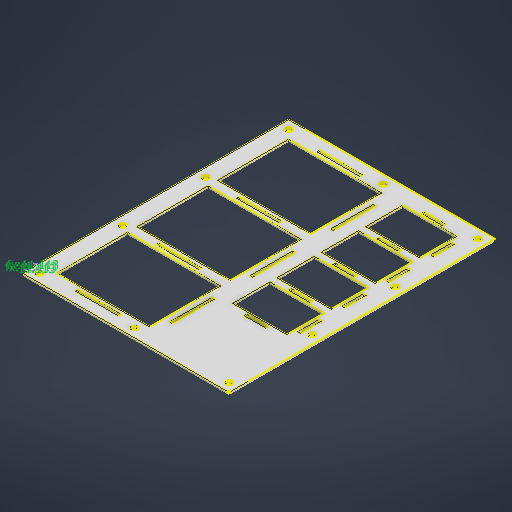
# Autodesk Inventor part: SignFace
Saved by Autodesk Inventor 2026 (Build 300175000, 175)
## iProperties
Created: 2025-05-16
Part Number: SignFace
Material: Generic
Document SubType Name: Modeling
Designer: Riley
Density: 1 g/cm^3
Appearance: Default
Author: Riley
Autodesk Inventor part; units mm, degrees
ref_plane "YZ Plane" through (0, 0, 0) normal (1, 0, 0) x (0, 1, 0)
ref_plane "XZ Plane" through (0, 0, 0) normal (0, 1, 0) x (-1, 0, 0)
ref_plane "XY Plane" through (0, 0, 0) normal (0, 0, 1) x (1, 0, 0)
sketch "Sketch1" plane through (0, 0, 0) normal (0, 1, 0) x (-1, 0, 0)
  line L0 (0, 0) -> (244, 0)
  line L1 (244, 0) -> (244, -314.35)
  line L2 (244, -314.35) -> (0, -314.35)
  line L3 (0, -314.35) -> (0, 0)
  line L4 (224, -20) -> (114, -20)
  line L5 (114, -20) -> (114, -104)
  line L6 (114, -104) -> (224, -104)
  line L7 (224, -104) -> (224, -20)
  line L8 (89, -294.35) -> (25, -294.35)
  line L9 (25, -294.35) -> (25, -250.35)
  line L10 (25, -250.35) -> (89, -250.35)
  line L11 (89, -250.35) -> (89, -294.35)
  line L12 (229.75, -107) -> (108.25, -107) construction
  line L13 (108.25, -107) -> (108.25, -17) construction
  line L14 (108.25, -17) -> (229.75, -17) construction
  line L15 (229.75, -17) -> (229.75, -107) construction
  line L16 (91.5, -248.75) -> (22.5, -248.75) construction
  line L17 (22.5, -248.75) -> (22.5, -295.95) construction
  line L18 (22.5, -295.95) -> (91.5, -295.95) construction
  line L19 (91.5, -295.95) -> (91.5, -248.75) construction
  line L20 (194.4, -108) -> (143.6, -108)
  line L21 (143.6, -108) -> (143.6, -111.175)
  line L22 (143.6, -111.175) -> (194.4, -111.175)
  line L23 (194.4, -111.175) -> (194.4, -108)
  line L24 (194.4, -16) -> (143.6, -16)
  line L25 (143.6, -16) -> (143.6, -12.825)
  line L26 (143.6, -12.825) -> (194.4, -12.825)
  line L27 (194.4, -12.825) -> (194.4, -16)
  line L28 (107.25, -36.6) -> (104.075, -36.6)
  line L29 (104.075, -36.6) -> (104.075, -87.4)
  line L30 (104.075, -87.4) -> (107.25, -87.4)
  line L31 (107.25, -87.4) -> (107.25, -36.6)
  line L32 (194.4, -206.35) -> (194.4, -203.175)
  line L33 (143.6, -203.175) -> (143.6, -206.35)
  line L34 (194.4, -203.175) -> (143.6, -203.175)
  line L35 (143.6, -206.35) -> (194.4, -206.35)
  line L36 (104.075, -182.575) -> (107.25, -182.575)
  line L37 (114, -115.175) -> (114, -199.175)
  line L38 (108.25, -202.175) -> (108.25, -112.175) construction
  line L39 (107.25, -182.575) -> (107.25, -131.775)
  line L40 (107.25, -131.775) -> (104.075, -131.775)
  line L41 (104.075, -131.775) -> (104.075, -182.575)
  line L42 (224, -115.175) -> (114, -115.175)
  line L43 (114, -199.175) -> (224, -199.175)
  line L44 (229.75, -202.175) -> (108.25, -202.175) construction
  line L45 (224, -199.175) -> (224, -115.175)
  line L46 (229.75, -112.175) -> (229.75, -202.175) construction
  line L47 (108.25, -112.175) -> (229.75, -112.175) construction
  line L48 (194.4, -301.525) -> (194.4, -298.35)
  line L49 (143.6, -298.35) -> (143.6, -301.525)
  line L50 (194.4, -298.35) -> (143.6, -298.35)
  line L51 (143.6, -301.525) -> (194.4, -301.525)
  line L52 (104.075, -277.75) -> (107.25, -277.75)
  line L53 (114, -210.35) -> (114, -294.35)
  line L54 (108.25, -297.35) -> (108.25, -207.35) construction
  line L55 (107.25, -277.75) -> (107.25, -226.95)
  line L56 (107.25, -226.95) -> (104.075, -226.95)
  line L57 (104.075, -226.95) -> (104.075, -277.75)
  line L58 (224, -210.35) -> (114, -210.35)
  line L59 (114, -294.35) -> (224, -294.35)
  line L60 (229.75, -297.35) -> (108.25, -297.35) construction
  line L61 (224, -294.35) -> (224, -210.35)
  line L62 (229.75, -207.35) -> (229.75, -297.35) construction
  line L63 (108.25, -207.35) -> (229.75, -207.35) construction
  line L64 (69.7, -247.75) -> (44.3, -247.75)
  line L65 (44.3, -247.75) -> (44.3, -244.575)
  line L66 (44.3, -244.575) -> (69.7, -244.575)
  line L67 (69.7, -244.575) -> (69.7, -247.75)
  line L68 (69.7, -296.95) -> (44.3, -296.95)
  line L69 (44.3, -296.95) -> (44.3, -300.125)
  line L70 (44.3, -300.125) -> (69.7, -300.125)
  line L71 (69.7, -300.125) -> (69.7, -296.95)
  line L72 (21.5, -259.65) -> (18.325, -259.65)
  line L73 (18.325, -259.65) -> (18.325, -285.05)
  line L74 (18.325, -285.05) -> (21.5, -285.05)
  line L75 (21.5, -285.05) -> (21.5, -259.65)
  line L76 (25, -241.975) -> (25, -197.975)
  line L77 (44.3, -195.375) -> (44.3, -192.2)
  line L78 (21.5, -207.275) -> (18.325, -207.275)
  line L79 (21.5, -232.675) -> (21.5, -207.275)
  line L80 (18.325, -207.275) -> (18.325, -232.675)
  line L81 (18.325, -232.675) -> (21.5, -232.675)
  line L82 (89, -241.975) -> (25, -241.975)
  line L83 (25, -197.975) -> (89, -197.975)
  line L84 (44.3, -192.2) -> (69.7, -192.2)
  line L85 (69.7, -195.375) -> (44.3, -195.375)
  line L86 (91.5, -196.375) -> (22.5, -196.375) construction
  line L87 (89, -197.975) -> (89, -241.975)
  line L88 (69.7, -192.2) -> (69.7, -195.375)
  line L89 (22.5, -196.375) -> (22.5, -243.575) construction
  line L90 (22.5, -243.575) -> (91.5, -243.575) construction
  line L91 (91.5, -243.575) -> (91.5, -196.375) construction
  line L92 (25, -189.6) -> (25, -145.6)
  line L93 (44.3, -143) -> (44.3, -139.825)
  line L94 (21.5, -154.9) -> (18.325, -154.9)
  line L95 (21.5, -180.3) -> (21.5, -154.9)
  line L96 (18.325, -154.9) -> (18.325, -180.3)
  line L97 (18.325, -180.3) -> (21.5, -180.3)
  line L98 (89, -189.6) -> (25, -189.6)
  line L99 (25, -145.6) -> (89, -145.6)
  line L100 (44.3, -139.825) -> (69.7, -139.825)
  line L101 (69.7, -143) -> (44.3, -143)
  line L102 (91.5, -144) -> (22.5, -144) construction
  line L103 (89, -145.6) -> (89, -189.6)
  line L104 (69.7, -139.825) -> (69.7, -143)
  line L105 (22.5, -144) -> (22.5, -191.2) construction
  line L106 (22.5, -191.2) -> (91.5, -191.2) construction
  line L107 (91.5, -191.2) -> (91.5, -144) construction
  line L108 (25, -137.225) -> (25, -93.225)
  line L109 (44.3, -90.625) -> (44.3, -87.45)
  line L110 (21.5, -102.525) -> (18.325, -102.525)
  line L111 (21.5, -127.925) -> (21.5, -102.525)
  line L112 (18.325, -102.525) -> (18.325, -127.925)
  line L113 (18.325, -127.925) -> (21.5, -127.925)
  line L114 (89, -137.225) -> (25, -137.225)
  line L115 (25, -93.225) -> (89, -93.225)
  line L116 (44.3, -87.45) -> (69.7, -87.45)
  line L117 (69.7, -90.625) -> (44.3, -90.625)
  line L118 (91.5, -91.625) -> (22.5, -91.625) construction
  line L119 (89, -93.225) -> (89, -137.225)
  line L120 (69.7, -87.45) -> (69.7, -90.625)
  line L121 (22.5, -91.625) -> (22.5, -138.825) construction
  line L122 (22.5, -138.825) -> (91.5, -138.825) construction
  line L123 (91.5, -138.825) -> (91.5, -91.625) construction
  circle A0 centre (234, -10) radius 3.5719
  circle A1 centre (234, -108.1167) radius 3.5719
  circle A2 centre (234, -206.2333) radius 3.5719
  circle A3 centre (234, -304.35) radius 3.5719
  circle A4 centre (122, -10) radius 3.5719
  circle A5 centre (10, -10) radius 3.5719
  circle A6 centre (10, -108.1167) radius 3.5719
  circle A7 centre (10, -206.2333) radius 3.5719
  circle A8 centre (10, -304.35) radius 3.5719
  circle A9 centre (122, -304.35) radius 3.5719
  point P0 (229.75, -62)
  point P1 (229.75, -157.175)
  point P2 (229.75, -252.35)
  dimension "d2" = 110
  dimension "d3" = 84
  dimension "d11" = 20
  dimension "d12" = 20
  dimension "d14" = 64
  dimension "d15" = 44
  dimension "d17" = 20
  dimension "d18" = 25
  dimension "d28" = 90
  dimension "d29" = 121.5
  dimension "d30" = 3
  dimension "d31" = 5.75
  dimension "d32" = 47.2
  dimension "d33" = 69
  dimension "d34" = 2.5
  dimension "d35" = 1.6
  dimension "d66" = 50.8
  dimension "d67" = 3.175
  dimension "d69" = 4
  dimension "d70" = 3.175
  dimension "d71" = 4
  dimension "d72" = 50.8
  dimension "d73" = 3.175
  dimension "d74" = 50.8
  dimension "d75" = 6.75
  dimension "d79" = 95.175
  dimension "d84" = 25.4
  dimension "d85" = 3.175
  dimension "d86" = 2.6
  dimension "d87" = 25.4
  dimension "d88" = 3.175
  dimension "d89" = 2.6
  dimension "d97" = 25.4
  dimension "d98" = 3.175
  dimension "d99" = 3.5
  dimension "d102" = 52.375
  dimension "d107" = 25
  dimension "d108" = 20
  dimension "d109" = 29.6
  dimension "d110" = 29.6
  dimension "d111" = 16.6
  dimension "d112" = 19.3
  dimension "d113" = 19.3
  dimension "d114" = 9.3
  dimension "d129" = 7.1437
  dimension "d130" = 10
  dimension "d131" = 10
  dimension "d132" = 314.35
  dimension "d133" = 244
  dimension "d136" = 98.1167
  dimension "d143" = 112
  dimension "d150" = 98.1167
  dimension "d157" = 112
  constraints: 248 end point, 22 parallel, 13 horizontal, 11 perpendicular, 10 centre point, 4 vertical, 2 collinear, 1 midpoint, 178 other
  measures "d2" distance of L6.end L5.end
  measures "d3" distance of L5.end L4.end
  measures "d11" distance between parallel lines of L1 L7
  measures "d12" distance between parallel lines of L0 L4
  measures "d14" distance of L9.end L10.end
  measures "d15" distance of L8.end L9.end
  measures "d17" distance between parallel lines of L2 L8
  measures "d18" distance between parallel lines of L3 L9
  measures "d28" distance between parallel lines of L12 L14
  measures "d29" distance from line of L13 point (229.75, -62)
  measures "d30" distance between parallel lines of L14 L4
  measures "d31" distance between parallel lines of L15 L7
  measures "d32" distance between parallel lines of L18 L16
  measures "d33" distance between parallel lines of L17 L19
  measures "d34" distance between parallel lines of L11 L19
  measures "d35" distance between parallel lines of L10 L16
  measures "d66" distance of L22.end L21.end
  measures "d67" distance of L21.end L20.end
  measures "d69" distance between parallel lines of L6 L20
  measures "d70" distance between parallel lines of L24 L26
  measures "d71" distance between parallel lines of L4 L24
  measures "d72" distance between parallel lines of L25 L27
  measures "d73" distance between parallel lines of L29 L31
  measures "d74" distance between parallel lines of L28 L30
  measures "d75" distance between parallel lines of L5 L31
  measures "d79" distance of L20.start L32.end
  measures "d84" distance between parallel lines of L65 L67
  measures "d85" distance between parallel lines of L66 L64
  measures "d86" distance between parallel lines of L10 L64
  measures "d87" distance between parallel lines of L69 L71
  measures "d88" distance between parallel lines of L68 L70
  measures "d89" distance between parallel lines of L8 L68
  measures "d97" distance between parallel lines of L74 L72
  measures "d98" distance between parallel lines of L75 L73
  measures "d99" distance between parallel lines of L9 L75
  measures "d102" distance of L9.end L76.end
  measures "d107" distance between parallel lines of L37 L119
  measures "d108" distance between parallel lines of L2 L59
  measures "d109" distance between parallel lines of L7 L27
  measures "d110" distance between parallel lines of L7 L23
  measures "d111" distance between parallel lines of L4 L28
  measures "d112" distance between parallel lines of L11 L71
  measures "d113" distance between parallel lines of L11 L67
  measures "d114" distance between parallel lines of L10 L72
  measures "d129" diameter of A0
  measures "d130" distance from line of L1 A0.centre
  measures "d131" distance from line of L0 A0.centre
  measures "d132" distance of L0.end L1.end
  measures "d133" distance of L1.end L2.end
  measures "d136" distance of A0.centre A1.centre
  measures "d143" distance of A0.centre A4.centre
  measures "d150" distance of A5.centre A6.centre
  measures "d157" distance of A3.centre A9.centre
extrude "Extrusion1" add sketch "Sketch1" along normal blind 3.175
sketch "Sketch3" plane through (0, 0, 0) normal (0, -1, 0) x (1, 0, 0)
  line L0 (0, -314.35) -> (-244, -314.35) projected
  line L1 (0, 0) -> (0, -314.35) projected
  line L2 (-244, 0) -> (0, 0) projected
  line L3 (-244, -314.35) -> (-244, 0) projected
  line L4 (-21.5, -102.525) -> (-21.5, -127.925) projected
  line L5 (-18.325, -102.525) -> (-21.5, -102.525) projected
  line L6 (-18.325, -127.925) -> (-18.325, -102.525) projected
  line L7 (-21.5, -127.925) -> (-18.325, -127.925) projected
  line L8 (-44.3, -90.625) -> (-44.3, -87.45) projected
  line L9 (-69.7, -90.625) -> (-44.3, -90.625) projected
  line L10 (-69.7, -87.45) -> (-69.7, -90.625) projected
  line L11 (-44.3, -87.45) -> (-69.7, -87.45) projected
  line L12 (-25, -137.225) -> (-25, -93.225) projected
  line L13 (-89, -137.225) -> (-25, -137.225) projected
  line L14 (-89, -93.225) -> (-89, -137.225) projected
  line L15 (-25, -93.225) -> (-89, -93.225) projected
  line L16 (-21.5, -154.9) -> (-21.5, -180.3) projected
  line L17 (-18.325, -154.9) -> (-21.5, -154.9) projected
  line L18 (-18.325, -180.3) -> (-18.325, -154.9) projected
  line L19 (-21.5, -180.3) -> (-18.325, -180.3) projected
  line L20 (-44.3, -143) -> (-44.3, -139.825) projected
  line L21 (-69.7, -143) -> (-44.3, -143) projected
  line L22 (-69.7, -139.825) -> (-69.7, -143) projected
  line L23 (-44.3, -139.825) -> (-69.7, -139.825) projected
  line L24 (-25, -189.6) -> (-25, -145.6) projected
  line L25 (-89, -189.6) -> (-25, -189.6) projected
  line L26 (-89, -145.6) -> (-89, -189.6) projected
  line L27 (-25, -145.6) -> (-89, -145.6) projected
  line L28 (-21.5, -207.275) -> (-21.5, -232.675) projected
  line L29 (-18.325, -207.275) -> (-21.5, -207.275) projected
  line L30 (-18.325, -232.675) -> (-18.325, -207.275) projected
  line L31 (-21.5, -232.675) -> (-18.325, -232.675) projected
  line L32 (-44.3, -195.375) -> (-44.3, -192.2) projected
  line L33 (-69.7, -195.375) -> (-44.3, -195.375) projected
  line L34 (-69.7, -192.2) -> (-69.7, -195.375) projected
  line L35 (-44.3, -192.2) -> (-69.7, -192.2) projected
  line L36 (-25, -241.975) -> (-25, -197.975) projected
  line L37 (-89, -241.975) -> (-25, -241.975) projected
  line L38 (-89, -197.975) -> (-89, -241.975) projected
  line L39 (-25, -197.975) -> (-89, -197.975) projected
  line L40 (-21.5, -259.65) -> (-21.5, -285.05) projected
  line L41 (-18.325, -259.65) -> (-21.5, -259.65) projected
  line L42 (-18.325, -285.05) -> (-18.325, -259.65) projected
  line L43 (-21.5, -285.05) -> (-18.325, -285.05) projected
  line L44 (-69.7, -296.95) -> (-69.7, -300.125) projected
  line L45 (-44.3, -296.95) -> (-69.7, -296.95) projected
  line L46 (-44.3, -300.125) -> (-44.3, -296.95) projected
  line L47 (-69.7, -300.125) -> (-44.3, -300.125) projected
  line L48 (-69.7, -247.75) -> (-44.3, -247.75) projected
  line L49 (-69.7, -244.575) -> (-69.7, -247.75) projected
  line L50 (-44.3, -244.575) -> (-69.7, -244.575) projected
  line L51 (-44.3, -247.75) -> (-44.3, -244.575) projected
  line L52 (-114, -210.35) -> (-224, -210.35) projected
  line L53 (-114, -294.35) -> (-114, -210.35) projected
  line L54 (-224, -294.35) -> (-114, -294.35) projected
  line L55 (-224, -210.35) -> (-224, -294.35) projected
  line L56 (-104.075, -277.75) -> (-104.075, -226.95) projected
  line L57 (-107.25, -277.75) -> (-104.075, -277.75) projected
  line L58 (-107.25, -226.95) -> (-107.25, -277.75) projected
  line L59 (-104.075, -226.95) -> (-107.25, -226.95) projected
  line L60 (-194.4, -301.525) -> (-143.6, -301.525) projected
  line L61 (-194.4, -298.35) -> (-194.4, -301.525) projected
  line L62 (-143.6, -298.35) -> (-194.4, -298.35) projected
  line L63 (-143.6, -301.525) -> (-143.6, -298.35) projected
  line L64 (-114, -115.175) -> (-224, -115.175) projected
  line L65 (-114, -199.175) -> (-114, -115.175) projected
  line L66 (-224, -199.175) -> (-114, -199.175) projected
  line L67 (-224, -115.175) -> (-224, -199.175) projected
  line L68 (-104.075, -182.575) -> (-104.075, -131.775) projected
  line L69 (-107.25, -182.575) -> (-104.075, -182.575) projected
  line L70 (-107.25, -131.775) -> (-107.25, -182.575) projected
  line L71 (-104.075, -131.775) -> (-107.25, -131.775) projected
  line L72 (-194.4, -206.35) -> (-143.6, -206.35) projected
  line L73 (-194.4, -203.175) -> (-194.4, -206.35) projected
  line L74 (-143.6, -203.175) -> (-194.4, -203.175) projected
  line L75 (-143.6, -206.35) -> (-143.6, -203.175) projected
  line L76 (-107.25, -36.6) -> (-107.25, -87.4) projected
  line L77 (-104.075, -36.6) -> (-107.25, -36.6) projected
  line L78 (-104.075, -87.4) -> (-104.075, -36.6) projected
  line L79 (-107.25, -87.4) -> (-104.075, -87.4) projected
  line L80 (-194.4, -16) -> (-143.6, -16) projected
  line L81 (-194.4, -12.825) -> (-194.4, -16) projected
  line L82 (-143.6, -12.825) -> (-194.4, -12.825) projected
  line L83 (-143.6, -16) -> (-143.6, -12.825) projected
  line L84 (-194.4, -108) -> (-194.4, -111.175) projected
  line L85 (-143.6, -108) -> (-194.4, -108) projected
  line L86 (-143.6, -111.175) -> (-143.6, -108) projected
  line L87 (-194.4, -111.175) -> (-143.6, -111.175) projected
  line L88 (-89, -294.35) -> (-25, -294.35) projected
  line L89 (-89, -250.35) -> (-89, -294.35) projected
  line L90 (-25, -250.35) -> (-89, -250.35) projected
  line L91 (-25, -294.35) -> (-25, -250.35) projected
  line L92 (-224, -20) -> (-224, -104) projected
  line L93 (-114, -20) -> (-224, -20) projected
  line L94 (-114, -104) -> (-114, -20) projected
  line L95 (-224, -104) -> (-114, -104) projected
extrude "Extrusion2" [suppressed]
sketch "Sketch4" plane through (0, 3.175, 0) normal (0, 1, 0) x (1, 0, 0)
  line L0 (0, 314.35) -> (-244, 314.35) projected
  line L1 (-244, 314.35) -> (-244, 0) projected
  line L2 (-244, 0) -> (0, 0) projected
  line L3 (0, 0) -> (0, 314.35) projected
  circle A0 centre (-122, 304.35) radius 3.5719 projected
  circle A1 centre (-10, 206.2333) radius 3.5719 projected
  circle A2 centre (-10, 108.1167) radius 3.5719 projected
  circle A3 centre (-10, 10) radius 3.5719 projected
  circle A4 centre (-122, 10) radius 3.5719 projected
  circle A5 centre (-234, 304.35) radius 3.5719 projected
  circle A6 centre (-234, 206.2333) radius 3.5719 projected
  circle A7 centre (-234, 108.1167) radius 3.5719 projected
  circle A8 centre (-234, 10) radius 3.5719 projected
  circle A9 centre (-10, 304.35) radius 3.5719 projected
  line L4 (-21.5, 102.525) -> (-21.5, 127.925) projected
  line L5 (-21.5, 127.925) -> (-18.325, 127.925) projected
  line L6 (-18.325, 127.925) -> (-18.325, 102.525) projected
  line L7 (-18.325, 102.525) -> (-21.5, 102.525) projected
  line L8 (-44.3, 90.625) -> (-44.3, 87.45) projected
  line L9 (-44.3, 87.45) -> (-69.7, 87.45) projected
  line L10 (-69.7, 87.45) -> (-69.7, 90.625) projected
  line L11 (-69.7, 90.625) -> (-44.3, 90.625) projected
  line L12 (-25, 137.225) -> (-25, 93.225) projected
  line L13 (-25, 93.225) -> (-89, 93.225) projected
  line L14 (-89, 93.225) -> (-89, 137.225) projected
  line L15 (-89, 137.225) -> (-25, 137.225) projected
  line L16 (-21.5, 154.9) -> (-21.5, 180.3) projected
  line L17 (-21.5, 180.3) -> (-18.325, 180.3) projected
  line L18 (-18.325, 180.3) -> (-18.325, 154.9) projected
  line L19 (-18.325, 154.9) -> (-21.5, 154.9) projected
  line L20 (-44.3, 143) -> (-44.3, 139.825) projected
  line L21 (-44.3, 139.825) -> (-69.7, 139.825) projected
  line L22 (-69.7, 139.825) -> (-69.7, 143) projected
  line L23 (-69.7, 143) -> (-44.3, 143) projected
  line L24 (-25, 189.6) -> (-25, 145.6) projected
  line L25 (-25, 145.6) -> (-89, 145.6) projected
  line L26 (-89, 145.6) -> (-89, 189.6) projected
  line L27 (-89, 189.6) -> (-25, 189.6) projected
  line L28 (-21.5, 207.275) -> (-21.5, 232.675) projected
  line L29 (-21.5, 232.675) -> (-18.325, 232.675) projected
  line L30 (-18.325, 232.675) -> (-18.325, 207.275) projected
  line L31 (-18.325, 207.275) -> (-21.5, 207.275) projected
  line L32 (-44.3, 195.375) -> (-44.3, 192.2) projected
  line L33 (-44.3, 192.2) -> (-69.7, 192.2) projected
  line L34 (-69.7, 192.2) -> (-69.7, 195.375) projected
  line L35 (-69.7, 195.375) -> (-44.3, 195.375) projected
  line L36 (-25, 241.975) -> (-25, 197.975) projected
  line L37 (-25, 197.975) -> (-89, 197.975) projected
  line L38 (-89, 197.975) -> (-89, 241.975) projected
  line L39 (-89, 241.975) -> (-25, 241.975) projected
  line L40 (-21.5, 259.65) -> (-21.5, 285.05) projected
  line L41 (-21.5, 285.05) -> (-18.325, 285.05) projected
  line L42 (-18.325, 285.05) -> (-18.325, 259.65) projected
  line L43 (-18.325, 259.65) -> (-21.5, 259.65) projected
  line L44 (-69.7, 296.95) -> (-69.7, 300.125) projected
  line L45 (-69.7, 300.125) -> (-44.3, 300.125) projected
  line L46 (-44.3, 300.125) -> (-44.3, 296.95) projected
  line L47 (-44.3, 296.95) -> (-69.7, 296.95) projected
  line L48 (-69.7, 247.75) -> (-44.3, 247.75) projected
  line L49 (-44.3, 247.75) -> (-44.3, 244.575) projected
  line L50 (-44.3, 244.575) -> (-69.7, 244.575) projected
  line L51 (-69.7, 244.575) -> (-69.7, 247.75) projected
  line L52 (-114, 210.35) -> (-224, 210.35) projected
  line L53 (-224, 210.35) -> (-224, 294.35) projected
  line L54 (-224, 294.35) -> (-114, 294.35) projected
  line L55 (-114, 294.35) -> (-114, 210.35) projected
  line L56 (-104.075, 277.75) -> (-104.075, 226.95) projected
  line L57 (-104.075, 226.95) -> (-107.25, 226.95) projected
  line L58 (-107.25, 226.95) -> (-107.25, 277.75) projected
  line L59 (-107.25, 277.75) -> (-104.075, 277.75) projected
  line L60 (-194.4, 301.525) -> (-143.6, 301.525) projected
  line L61 (-143.6, 301.525) -> (-143.6, 298.35) projected
  line L62 (-143.6, 298.35) -> (-194.4, 298.35) projected
  line L63 (-194.4, 298.35) -> (-194.4, 301.525) projected
  line L64 (-114, 115.175) -> (-224, 115.175) projected
  line L65 (-224, 115.175) -> (-224, 199.175) projected
  line L66 (-224, 199.175) -> (-114, 199.175) projected
  line L67 (-114, 199.175) -> (-114, 115.175) projected
  line L68 (-104.075, 182.575) -> (-104.075, 131.775) projected
  line L69 (-104.075, 131.775) -> (-107.25, 131.775) projected
  line L70 (-107.25, 131.775) -> (-107.25, 182.575) projected
  line L71 (-107.25, 182.575) -> (-104.075, 182.575) projected
  line L72 (-194.4, 206.35) -> (-143.6, 206.35) projected
  line L73 (-143.6, 206.35) -> (-143.6, 203.175) projected
  line L74 (-143.6, 203.175) -> (-194.4, 203.175) projected
  line L75 (-194.4, 203.175) -> (-194.4, 206.35) projected
  line L76 (-107.25, 36.6) -> (-107.25, 87.4) projected
  line L77 (-107.25, 87.4) -> (-104.075, 87.4) projected
  line L78 (-104.075, 87.4) -> (-104.075, 36.6) projected
  line L79 (-104.075, 36.6) -> (-107.25, 36.6) projected
  line L80 (-194.4, 16) -> (-143.6, 16) projected
  line L81 (-143.6, 16) -> (-143.6, 12.825) projected
  line L82 (-143.6, 12.825) -> (-194.4, 12.825) projected
  line L83 (-194.4, 12.825) -> (-194.4, 16) projected
  line L84 (-194.4, 108) -> (-194.4, 111.175) projected
  line L85 (-194.4, 111.175) -> (-143.6, 111.175) projected
  line L86 (-143.6, 111.175) -> (-143.6, 108) projected
  line L87 (-143.6, 108) -> (-194.4, 108) projected
  line L88 (-89, 294.35) -> (-25, 294.35) projected
  line L89 (-25, 294.35) -> (-25, 250.35) projected
  line L90 (-25, 250.35) -> (-89, 250.35) projected
  line L91 (-89, 250.35) -> (-89, 294.35) projected
  line L92 (-224, 20) -> (-224, 104) projected
  line L93 (-224, 104) -> (-114, 104) projected
  line L94 (-114, 104) -> (-114, 20) projected
  line L95 (-114, 20) -> (-224, 20) projected
  line L96 (-250.7123, 8.394) -> (-250.7123, 14.8414)
  line L97 (-250.7123, 14.8414) -> (-244.8261, 17.8207)
  line L98 (-244.8261, 17.8207) -> (-239.5998, 14.4585)
  line L99 (-239.5998, 14.4585) -> (-239.5998, 8.0111)
  line L100 (-239.5998, 8.0111) -> (-245.486, 5.0318)
  line L101 (-245.486, 5.0318) -> (-250.7123, 8.394)
  dimension "d162" = 11.1125
  dimension "d163" = 11.1125
  dimension "d164" = 11.1125
  constraints: 12 end point, 4 parallel, 1 vertical
  measures "d162" distance between parallel lines of L99 L96
  measures "d163" distance between parallel lines of L98 L101
  measures "d164" distance between parallel lines of L97 L100
equation "\"d12\" = d11"
equation "\"d17\" = d11"
equation "\"d30\" = -0.5 * d3 + 0.5 * d28"
equation "\"d31\" = -0.5 * d2 + 0.5 * d29"
equation "\"d34\" = -0.5 * d14 + 0.5 * d33"
equation "\"d35\" = -0.5 * d15 + 0.5 * d32"
equation "\"d66\" = d72"
equation "\"d70\" = d67"
equation "\"d71\" = d69"
equation "\"d73\" = d67"
equation "\"d74\" = d72"
equation "\"d79\" = d67 + d3 + 2 * d69"
equation "\"d84\" = d87"
equation "\"d85\" = d67"
equation "\"d88\" = d85"
equation "\"d89\" = d86"
equation "\"d97\" = d87"
equation "\"d98\" = d85"
equation "\"d102\" = d85 + d15 + 2 * d86"
equation "\"d108\" = d11"
equation "\"d109\" = -0.5 * d72 + 0.5 * d2"
equation "\"d110\" = d109"
equation "\"d111\" = -0.5 * d74 + 0.5 * d3"
equation "\"d112\" = -0.5 * d87 + 0.5 * d14"
equation "\"d113\" = d112"
equation "\"d114\" = -0.5 * d97 + 0.5 * d15"
body "Solid1"
